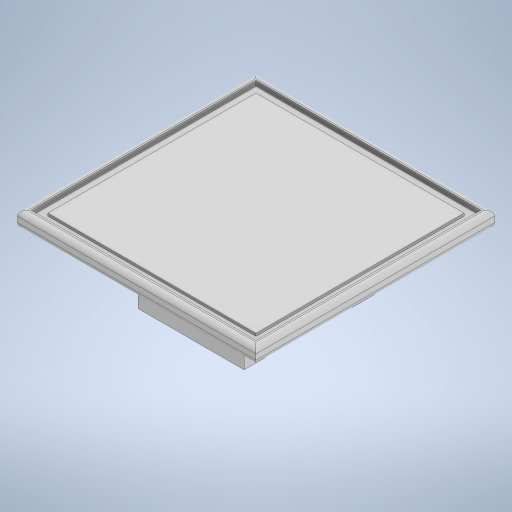
# Autodesk Inventor part: OV-PAM_n_4_bottom
Saved by Autodesk Inventor 2024 (Build 280153000, 153)
## iProperties
Created: 2023-08-31
Part Number: OV-PAM_n_4_bottom
Material: 일반
Document SubType Name: Modeling
Designer: jsw
Density: 1 g/cm^3
Appearance: 기본값
Author: jsw
Autodesk Inventor part; units mm, degrees
ref_plane "YZ Plane" through (0, 0, 0) normal (1, 0, 0) x (0, 1, 0)
ref_plane "XZ Plane" through (0, 0, 0) normal (0, 1, 0) x (-1, 0, 0)
ref_plane "XY Plane" through (0, 0, 0) normal (0, 0, 1) x (1, 0, 0)
sketch "스케치1" plane through (0, 0, 0) normal (0, 1, 0) x (-1, 0, 0)
  line L0 (-24.9446, -24.9446) -> (24.9446, -24.9446)
  line L1 (24.9446, -24.9446) -> (24.9446, 24.9446)
  line L2 (24.9446, 24.9446) -> (-24.9446, 24.9446)
  line L3 (-24.9446, 24.9446) -> (-24.9446, -24.9446)
  line L4 (-24.9446, -24.9446) -> (24.9446, 24.9446) construction
  line L5 (24.9446, -24.9446) -> (-24.9446, 24.9446) construction
  line L6 (-28.1446, -28.1446) -> (28.1446, -28.1446)
  line L7 (28.1446, -28.1446) -> (28.1446, 28.1446)
  line L8 (28.1446, 28.1446) -> (-28.1446, 28.1446)
  line L9 (-28.1446, 28.1446) -> (-28.1446, -28.1446)
  line L10 (-28.1446, -28.1446) -> (28.1446, 28.1446) construction
  line L11 (28.1446, -28.1446) -> (-28.1446, 28.1446) construction
  point P0 (0, 0)
  dimension "d0" = 70.554
  dimension "d1" = 3.2
  constraints: 24 end point, 4 midpoint, 4 parallel, 4 perpendicular, 2 horizontal
  measures "d0" distance of L2.end L0.end
  measures "d1" distance between parallel lines of L1 L7
extrude "돌출1" add sketch "스케치1" along normal blind 3.7 contours L3 L2 L1 L0 | L9 L8 L7 L6
sketch "스케치2" plane through (0, 3.7, 0) normal (0, 1, 0) x (1, 0, 0)
  line L0 (-28.1446, 28.1446) -> (-28.1446, -28.1446) projected
  line L1 (-28.1446, -28.1446) -> (28.1446, -28.1446) projected
  line L2 (28.1446, -28.1446) -> (28.1446, 28.1446) projected
  line L3 (28.1446, 28.1446) -> (-28.1446, 28.1446) projected
  line L4 (26.5446, 26.5446) -> (-26.5446, 26.5446)
  line L5 (-26.5446, 26.5446) -> (-26.5446, -26.5446)
  line L6 (-26.5446, -26.5446) -> (26.5446, -26.5446)
  line L7 (26.5446, -26.5446) -> (26.5446, 26.5446)
  line L8 (26.5446, 26.5446) -> (-26.5446, -26.5446) construction
  line L9 (-26.5446, 26.5446) -> (26.5446, -26.5446) construction
  line L10 (24.5446, 24.5446) -> (-24.5446, 24.5446)
  line L11 (-24.5446, 24.5446) -> (-24.5446, -24.5446)
  line L12 (-24.5446, -24.5446) -> (24.5446, -24.5446)
  line L13 (24.5446, -24.5446) -> (24.5446, 24.5446)
  line L14 (24.5446, 24.5446) -> (-24.5446, -24.5446) construction
  line L15 (-24.5446, 24.5446) -> (24.5446, -24.5446) construction
  point P0 (0, 0)
  point P1 (0, 28.1446)
  point P2 (-28.1446, 0)
  dimension "d4" = 1.6
  dimension "d5" = 2
  constraints: 24 end point, 6 midpoint, 4 parallel, 3 perpendicular, 2 horizontal, 1 horizontal alignment, 1 point on line, 1 vertical alignment
  measures "d4" distance between parallel lines of L5 L0
  measures "d5" distance between parallel lines of L11 L5
extrude "돌출2" cut sketch "스케치2" against normal blind 1.2 contours L7 L6 L5 L4 | L13 L12 L11 L10
sketch "스케치3" plane through (0, 2.5, 0) normal (0, 1, 0) x (1, 0, 0)
  line L0 (24.5446, 24.5446) -> (-24.5446, 24.5446)
  line L1 (-24.5446, 24.5446) -> (-24.5446, -24.5446)
  line L2 (-24.5446, -24.5446) -> (24.5446, -24.5446)
  line L3 (24.5446, -24.5446) -> (24.5446, 24.5446)
  line L4 (24.5446, 24.5446) -> (-24.5446, -24.5446) construction
  line L5 (-24.5446, 24.5446) -> (24.5446, -24.5446) construction
  line L6 (-26.5446, -26.5446) -> (-26.5446, 26.5446) projected
  point P0 (0, 0)
  dimension "d8" = 2
  constraints: 12 end point, 2 midpoint, 2 parallel, 2 perpendicular, 1 horizontal
  measures "d8" distance between parallel lines of L1 L6
extrude "돌출3" add sketch "스케치3" along normal blind 0.6
fillet "모깎기1" radius 1.2 8 edges at (0, 3.7, 28.1446) (28.1446, 3.7, 0) (0, 3.7, -28.1446) (-28.1446, 3.7, 0) (-28.1446, 0, 0) (0, 0, 28.1446) (28.1446, 0, 0) (0, 0, -28.1446)
sketch "스케치10" plane through (0, 0, 0) normal (0, -1, 0) x (1, 0, 0)
  line L0 (-12.5, 10.3) -> (12.5, 10.3)
  line L1 (12.5, 10.3) -> (12.5, 15.3)
  line L2 (12.5, 15.3) -> (-12.5, 15.3)
  line L3 (-12.5, 15.3) -> (-12.5, 10.3)
  line L4 (-12.5, 10.3) -> (12.5, 15.3) construction
  line L5 (12.5, 10.3) -> (-12.5, 15.3) construction
  line L6 (0, 0) -> (6.1954, 0)
  line L7 (-12.5, -10.3) -> (12.5, -10.3)
  line L8 (12.5, -10.3) -> (12.5, -15.3)
  line L9 (12.5, -15.3) -> (-12.5, -15.3)
  line L10 (-12.5, -15.3) -> (-12.5, -10.3)
  line L11 (-12.5, -10.3) -> (12.5, -15.3) construction
  line L12 (12.5, -10.3) -> (-12.5, -15.3) construction
  point P0 (0, 12.8)
  point P1 (0, -12.8)
  dimension "d51" = 25
  dimension "d52" = 5
  dimension "d53" = 10.3
  constraints: 26 end point, 5 symmetric about line, 2 horizontal, 2 midpoint, 2 parallel, 1 perpendicular, 1 vertical alignment
  measures "d51" distance of L2.end L1.end
  measures "d52" distance of L0.end L1.end
  measures "d53" distance from line of L6.start L0
extrude "돌출7" add sketch "스케치10" along normal blind 15
sketch "스케치11" plane through (12.5, 0, -15.3) normal (0, 0, -1) x (-1, 0, 0)
  circle A0 centre (17.5, -7.5) radius 1.25
  line L0 (-14.4446, 0) -> (39.4446, 0) projected
  line L1 (12.5, 0) -> (12.5, -4.6677)
  circle A1 centre (7.5, -7.5) radius 1.25
  dimension "d56" = 2.5
  dimension "d57" = 7.5
  dimension "d58" = 5
  constraints: 2 centre point, 2 end point, 1 midpoint, 1 symmetric about line, 1 vertical, 1 other
  measures "d56" diameter of A0
  measures "d57" distance from line of A0.centre L0
  measures "d58" horizontal distance of L1.start A0.centre
extrude "돌출8" cut sketch "스케치11" against normal up to surface (30.6 mm away)
equation "\"d39\" = 55deg"
